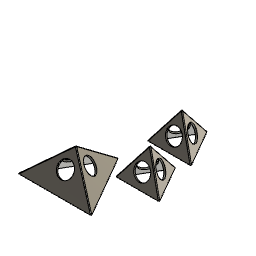
Painters tripod v5 (Autodesk Fusion 360 design; units mm, degrees)
Autodesk Fusion 360 part; units mm, degrees
sketch "bottom contour" plane through (0, 0, 0) normal (0, 0, 1) x (1, 0, 0) in component "tripod"
  line L0 (0, 0) -> (34.641, 60)
  line L1 (34.641, 60) -> (69.282, 0)
  line L2 (69.282, 0) -> (0, 0)
  dimension "d1" = 60
  constraint coincident L0.start L2.end
  constraint horizontal L2
  constraint equal L0 L1
  constraint equal L1 L2
  measures "d1" vertical distance of L0.start L0.end
ref_plane "WorkPlane1" through (34.641, 30, 50) normal (0, 0, 1) x (1, 0, 0) in component "tripod"
sketch "Sketch2" plane through (0, 0, 50) normal (0, 0, 1) x (1, 0, 0) in component "tripod"
  line L0 (0, 0) -> (34.641, 60)
  line L1 (34.641, 60) -> (69.282, 0)
  line L2 (69.282, 0) -> (0, 0)
  line L3 (34.641, 60) -> (34.641, 0) construction
  line L4 (51.9615, 30) -> (0, 0) construction
  point P0 (34.641, 20)
  constraint coincident L0.end L1.start
  constraint midpoint L2 L3.end
  constraint coincident L1 L4.start
  constraint perpendicular L1 L4
  constraint coincident L0.start L2.end
  constraint coincident L4 P0
  constraint coincident L3 P0
loft "Loft1" add profiles "bottom contour" section 1 section 2 point at (34.641, 20, 50) makes body 1 in component "tripod"
shell "Shell1" thickness 2.5 removed faces 1 at (34.641, 20, 0) on bodies 1 in component "tripod"
sketch "Sketch3" plane through (0, 0, 0) normal (0, -0.928477, 0.371391) x (1, 0, 0) in component "tripod"
  line L0 (0, 0) -> (69.282, 0)
  line L1 (69.282, 0) -> (34.641, 53.8516)
  line L2 (34.641, 53.8516) -> (0, 0)
  line L3 (34.641, 53.8516) -> (34.641, 0) construction
  line L4 (50.0157, 29.9507) -> (0, 0) construction
  circle A0 centre (34.641, 20.744) radius 12.5
  dimension "d4" = 25
  constraint coincident L1.end L2.start
  constraint midpoint L0 L3.end
  constraint coincident L1 L4.start
  constraint coincident L0.start L2.end
  constraint coincident L3 A0.centre
  constraint coincident L4 A0.centre
  measures "d4" diameter of A0
extrude "Extrude1" cut sketch "Sketch3" against normal blind 8 contours A0 bodies 1 in component "tripod"
pattern_circular "C-Pattern1" count 3 over 360 about axis through (34.641, 20, 75) along (0, 0, -1) of "Extrude1" in component "tripod"
fillet "Fillet1" radius 1 3 edges at (51.9615, 10, 25) (34.641, 40, 25) (17.3205, 10, 25) on bodies 1 in component "tripod"
sketch "bottom contour (2)" plane through (0, 0, 0) normal (0, 0, 1) x (1, 0, 0) in component "100mm tripod"
  line L0 (0, 0) -> (57.735, 100)
  line L1 (57.735, 100) -> (115.4701, 0)
  line L2 (115.4701, 0) -> (0, 0)
  dimension "d1_1" = 100
  constraint coincident L0.start L2.end
  constraint horizontal L2
  constraint equal L0 L1
  constraint equal L1 L2
  measures "d1_1" vertical distance of L0.start L0.end
ref_plane "WorkPlane1" through (57.735, 50, 50) normal (0, 0, 1) x (1, 0, 0) in component "100mm tripod"
sketch "Sketch2 (2)" plane through (0, 0, 50) normal (0, 0, 1) x (1, 0, 0) in component "100mm tripod"
  line L0 (0, 0) -> (57.735, 100)
  line L1 (57.735, 100) -> (115.4701, 0)
  line L2 (115.4701, 0) -> (0, 0)
  line L3 (57.735, 100) -> (57.735, 0) construction
  line L4 (86.6025, 50) -> (0, 0) construction
  point P0 (57.735, 33.3333)
  constraint coincident L0.end L1.start
  constraint midpoint L2 L3.end
  constraint coincident L1 L4.start
  constraint perpendicular L1 L4
  constraint coincident L0.start L2.end
  constraint coincident L4 P0
  constraint coincident L3 P0
loft "Loft1'" add profiles "bottom contour (2)" section 1 section 2 point at (57.735, 33.3333, 50) separate body makes body 2 in component "100mm tripod"
shell "Shell1'" thickness 2.5 removed faces 1 at (57.735, 33.3333, 0) on bodies 2 in component "100mm tripod"
sketch "Sketch3 (2)" plane through (0, 0, 0) normal (0, -0.83205, 0.5547) x (1, 0, 0) in component "100mm tripod"
  line L0 (0, 0) -> (115.4701, 0)
  line L1 (115.4701, 0) -> (57.735, 60.0925)
  line L2 (57.735, 60.0925) -> (0, 0)
  line L3 (57.735, 60.0925) -> (57.735, 0) construction
  line L4 (76.5492, 40.5101) -> (0, 0) construction
  circle A0 centre (57.735, 30.5536) radius 12.5
  dimension "d4_1" = 25
  constraint coincident L1.end L2.start
  constraint midpoint L0 L3.end
  constraint coincident L1 L4.start
  constraint coincident L0.start L2.end
  constraint coincident L3 A0.centre
  constraint coincident L4 A0.centre
  measures "d4_1" diameter of A0
extrude "Extrude1'" cut sketch "Sketch3 (2)" against normal blind 8 contours A0 bodies 2 in component "100mm tripod"
pattern_circular "C-Pattern1'" count 3 over 360 about axis through (57.735, 33.3333, 125) along (0, 0, -1) of "Extrude1'" in component "100mm tripod"
fillet "Fillet1'" radius 1 3 edges at (86.6025, 16.6667, 25) (57.735, 66.6667, 25) (28.8675, 16.6667, 25) on bodies 2 in component "100mm tripod"
component "tripod" placed x (1, 0, 0) y (0, 1, 0) z (0, 0, 1) at (0, 0, 0)
component "tripod" placed x (1, 0, 0) y (0, 1, 0) z (0, 0, 1) at (0, 70, 0)
component "100mm tripod" placed x (1, 0, 0) y (0, 1, 0) z (0, 0, 1) at (-62.0568, -124.2943, 7.7625)
